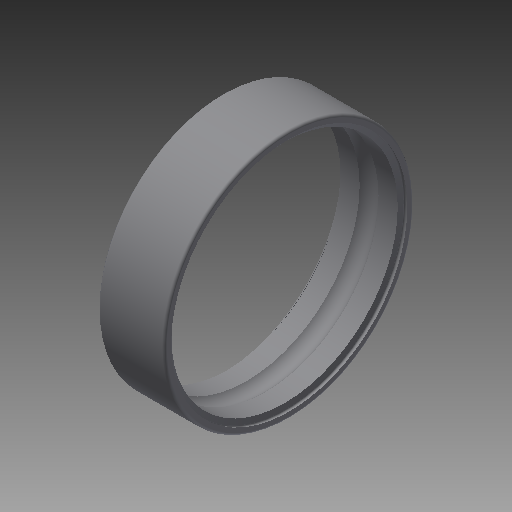
# Autodesk Inventor part: W 61700 X-2RS1_PART2
Saved by Autodesk Inventor 2018.3 (Build 223284000, 284)
## iProperties
Category: PARTsolutions
Company: SKF
Created: 2018-07-22
Part Number: W 61700 X-2RS1_PART2
Material: Generic
Catalog Web Link: www.cadenas.de
Description: -Deep groove ball bearings, stainless steel, single row
Vendor: SKF
Document SubType Name: Modeling
Designer: psadmin
Manufacturer: SKF
Mass: 0.109499 g
Surface Area: 4.29103 cm^2
Volume: 0.109499 cm^3
Density: 1 g/cm^3
Appearance: PSOLRGB-175-175-175
PSOL_IDENT_0: {$CADENAS_DATA\23d-libs\skf\bearings_units_and_housings\ball_bearings\deep_groove_ball_bearings\deep
PSOL_IDENT_1: _groove_ball_bearings_stainless_steel\bb1_004_104.prj},207 {VTYP=3D},{NB=W 61700 X-2RS1_PART2},{LINA=
PSOL_IDENT_2: W 61700 X-2RS1_PART2},{NN=BB1_004_104_PART2},{NOPRJ=TRUE},{DATE=13.07.2018 14:28:03},{GEOMDATE=26.07
PSOL_IDENT_3: .2017 12:34:56},{VERSION=},{LINEID=79600},{WBVAR=},{WBNUMERIC=}  {NB=W 61700 X-2RS1_PART2},{LINA=W 6
PSOL_IDENT_4: 1700 X-2RS1_PART2},{KT=DUMMY},{PRODUCTID=},{DESIGNATION=W 61700 X-2RS1},{DD=10.000},{D=15.000},{B=4.
PSOL_IDENT_5: 000},{DD1=11.210},{DD2=MIN},{D1=13.600},{D2=14.200},{R12A=0.150},{LOAD1=0.488},{LOAD2=0.220},{LOAD3=
PSOL_IDENT_6: 0.009},{SPEED1=24000},{SPEED2=},{MASS=0.002},{PITCH=12.490},{DW=1.588},{Z=11.000},{II=1.000},{TYPEID=
PSOL_IDENT_7: MIN},{YALG=5.605},{HALG=0.605},{HELP=0.7},{HELP2=0.4},{YALG1=6.8},{HALG1=0.7},{TAXONOMY=2},{DESIGN=d
PSOL_IDENT_8: gbbw2rs},{MAPPING=BCZ50,DESIGNATION|IRD01,DD|ORD10,D|BCW30,B|IRD30,DD1|ORD30,D1|ORD43,D2|IRD43,DD2|O
PSOL_IDENT_9: RR20,R12A|BCC02,LOAD1|BCC16,LOAD2|BCC12,LOAD3|BCC45,SPEED1|BCM01,MASS|BCD50,PITCH|RBD10,DW|BCN81,Z|B
PSOL_IDENT_10: CN80,II},{DESIGNLIST=dgbbw2z,dgbbw,dgbbw2rs},{SH=5.605},{SORT=DD},{RHELP=0.15},{PIM=W 61700 X-2RS1},
PSOL_IDENT_11: {R12=0.15},{HIDE=MIN}
NT: Deep groove ball bearings, stainless steel, single row
NB: W 61700 X-2RS1_PART2
NBSYN: $DESIGNATION._PART2
LINA: W 61700 X-2RS1_PART2
SUPPLIER: SKF
ARTICLENO: W 61700 X-2RS1_PART2
BOMINFO: W 61700 X-2RS1_PART2
CREATOR: CADENAS GmbH
Title: W 61700 X-2RS1_PART2
Author: Cadenas PARTsolutions
Comments: Deep groove ball bearings, stainless steel, single row
Autodesk Inventor part; units mm, degrees
ref_plane "YZ Plane" through (0, 0, 0) normal (1, 0, 0) x (0, 1, 0)
ref_plane "XZ Plane" through (0, 0, 0) normal (0, 1, 0) x (-1, 0, 0)
ref_plane "XY Plane" through (0, 0, 0) normal (0, 0, 1) x (1, 0, 0)
sketch "Sketch_4" plane through (0, 0, 0) normal (0, 0, 1) x (1, 0, 0)
  line L0 (50, 0) -> (-50, 0)
  line L1 (0, 7.1) -> (0.045, 7.1)
  arc A0 (0.225, 7.1) -> (0.045, 7.1) centre (0.135, 7.1) ccw
  line L2 (0.225, 7.1) -> (0.2779, 6.8)
  line L3 (0.2779, 6.8) -> (1.4322, 6.8)
  arc A1 (2.5678, 6.8) -> (1.4322, 6.8) centre (2, 6.245) ccw
  line L4 (2.5678, 6.8) -> (3.7221, 6.8)
  line L5 (3.7221, 6.8) -> (3.775, 7.1)
  arc A2 (3.955, 7.1) -> (3.775, 7.1) centre (3.865, 7.1) ccw
  line L6 (3.955, 7.1) -> (4, 7.1)
  line L7 (4, 7.1) -> (4, 7.35)
  arc A3 (4, 7.35) -> (3.85, 7.5) centre (3.85, 7.35) ccw
  line L8 (3.85, 7.5) -> (0.15, 7.5)
  arc A4 (0.15, 7.5) -> (0, 7.35) centre (0.15, 7.35) ccw
  line L9 (0, 7.35) -> (0, 7.1)
  constraints: 20 end point, 10 point on circle, 5 centre point
revolve "Revolution1" add sketch "Sketch_4" angle 360 about axis through (50, 0, 0) along (1, 0, 0)
body "Solid1"
